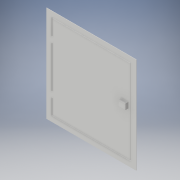
# Autodesk Inventor part: tetris backdoor
Saved by Autodesk Inventor 2017 (Build 210142000, 142)
## iProperties
Created: 2019-08-23
Part Number: tetris backdoor
Material: Generic
Document SubType Name: Modeling
Designer: EDMU0006
Density: 1 g/cm^3
Appearance: Default
Author: EDMU0006
Autodesk Inventor part; units mm, degrees
ref_plane "YZ Plane" through (0, 0, 0) normal (1, 0, 0) x (0, 1, 0)
ref_plane "XZ Plane" through (0, 0, 0) normal (0, 1, 0) x (-1, 0, 0)
ref_plane "XY Plane" through (0, 0, 0) normal (0, 0, 1) x (1, 0, 0)
sketch "Sketch1" plane through (0, 0, 0) normal (0, 0, 1) x (1, 0, 0)
  line L0 (-364.6328, 359.0746) -> (397.3672, 359.0746)
  line L1 (397.3672, 359.0746) -> (397.3672, -453.7254)
  line L2 (397.3672, -453.7254) -> (-364.6328, -453.7254)
  line L3 (-364.6328, -453.7254) -> (-364.6328, 359.0746)
  point P0 (0, 0)
  dimension "d0" = 762
  dimension "d1" = 812.8
  constraints: 8 end point, 2 parallel, 1 horizontal, 1 perpendicular
  measures "d0" distance of L1.end L2.end
  measures "d1" distance of L2.end L0.start
extrude "Extrusion1" add sketch "Sketch1" along normal blind 5.0038
sketch "Sketch2" plane through (0, 0, 5.0038) normal (0, 0, 1) x (1, 0, 0)
  line L0 (-313.8328, 308.2746) -> (346.5672, 308.2746)
  line L1 (346.5672, 308.2746) -> (346.5672, -402.9254)
  line L2 (346.5672, -402.9254) -> (-313.8328, -402.9254)
  line L3 (-313.8328, -402.9254) -> (-313.8328, 308.2746)
  line L4 (-364.6328, 359.0746) -> (397.3672, 359.0746) projected
  line L5 (-364.6328, -453.7254) -> (397.3672, -453.7254) projected
  line L6 (-364.6328, 359.0746) -> (-364.6328, -453.7254) projected
  line L7 (397.3672, -453.7254) -> (397.3672, 359.0746) projected
  line L8 (-318.9128, 313.3546) -> (351.6472, 313.3546)
  line L9 (351.6472, 313.3546) -> (351.6472, -408.0054)
  line L10 (351.6472, -408.0054) -> (-318.9128, -408.0054)
  line L11 (-318.9128, -408.0054) -> (-318.9128, 313.3546)
  point P0 (0, 0)
  dimension "d4" = 50.8
  dimension "d5" = 50.8
  dimension "d6" = 50.8
  dimension "d7" = 50.8
  dimension "d8" = 5.08
  dimension "d9" = 5.08
  dimension "d10" = 5.08
  dimension "d11" = 5.08
  constraints: 16 end point, 4 parallel, 2 horizontal, 2 perpendicular
  measures "d4" distance between parallel lines of L4 L0
  measures "d5" distance between parallel lines of L5 L2
  measures "d6" distance between parallel lines of L3 L6
  measures "d7" distance between parallel lines of L7 L1
  measures "d8" distance between parallel lines of L0 L8
  measures "d9" distance between parallel lines of L11 L3
  measures "d10" distance between parallel lines of L1 L9
  measures "d11" distance between parallel lines of L2 L10
extrude "Extrusion2" cut sketch "Sketch2" against normal blind 5.0038 contours L8 L9 L10 L11
sketch "Sketch3" plane through (-313.8328, -402.9254, 5.0038) normal (-1, 0, 0) x (0, 0, 1)
  line L0 (-5.0038, 762) -> (-5.0038, -50.8) projected
  line L1 (0, -50.8) -> (0, 762) projected
  line L2 (-5.0038, 577.2709) -> (0, 577.2709)
  line L3 (0, 577.2709) -> (0, 529.5342)
  line L4 (0, 529.5342) -> (-5.0038, 529.5342)
  line L5 (-5.0038, 529.5342) -> (-5.0038, 577.2709)
  line L6 (0, 174.3668) -> (0, 157.0851)
  line L7 (-5.0038, 157.0851) -> (-5.0038, 174.3668)
  line L8 (0, 0) -> (0, 711.2) projected
  line L9 (-5.0038, 174.3668) -> (0, 174.3668)
  line L10 (0, 174.3668) -> (0, 126.6402)
  line L11 (0, 126.6402) -> (-5.0038, 126.6402)
  line L12 (-5.0038, 126.6402) -> (-5.0038, 174.3668)
  point P0 (-5.0038, 402.9254)
  dimension "d16" = 47.7266
  constraints: 20 end point, 5 parallel, 5 point on line, 2 horizontal, 2 perpendicular
  measures "d16" distance of L9.end L10.end
extrude "Extrusion3" add sketch "Sketch3" along normal blind 5.0038 contours L2 L1 L4 L0 | L9 L1 L11 L0
sketch "Sketch4" plane through (0, 0, 5.0038) normal (0, 0, 1) x (1, 0, 0)
  line L0 (272.2721, 16.6455) -> (330.5312, 16.6455)
  line L1 (330.5312, 16.6455) -> (330.5312, -30.913)
  line L2 (330.5312, -30.913) -> (272.2721, -30.913)
  line L3 (272.2721, -30.913) -> (272.2721, 16.6455)
  point P0 (0, 0)
  constraints: 8 end point, 2 parallel, 1 horizontal, 1 perpendicular
extrude "Extrusion4" add sketch "Sketch4" along normal blind 25.4
fillet "Fillet1" radius 3.175 4 edges at (301.4017, 16.6455, 30.4038) (330.5312, -7.1338, 30.4038) (301.4017, -30.913, 30.4038) (272.2721, -7.1338, 30.4038)
body "Solid1"
